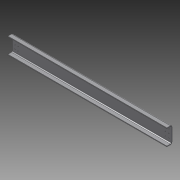
# Autodesk Inventor part: Base Back Bar
Saved by Autodesk Inventor 2012 (Build 160160000, 160)
## iProperties
Created: 2011-10-13
Part Number: Base Back Bar
Material: Default
Document SubType Name: Sheet Metal
Designer: Tushar
Density: 1 g/cm^3
Sheet Metal Rule: Default
Author: Tushar
Autodesk Inventor part; units mm, degrees
ref_plane "YZ Plane" through (0, 0, 0) normal (1, 0, 0) x (0, 1, 0)
ref_plane "XZ Plane" through (0, 0, 0) normal (0, 1, 0) x (-1, 0, 0)
ref_plane "XY Plane" through (0, 0, 0) normal (0, 0, 1) x (1, 0, 0)
sketch "Sketch2" plane through (0, 0, 0) normal (0, 0, 1) x (1, 0, 0)
  line L0 (-301.752, 25.273) -> (301.752, 25.273)
  line L1 (301.752, 25.273) -> (301.752, -25.273)
  line L2 (301.752, -25.273) -> (-301.752, -25.273)
  line L3 (-301.752, -25.273) -> (-301.752, 25.273)
  point P0 (0, 0)
  dimension "d0" = 301.752
  dimension "d1" = 301.752
  dimension "d2" = 25.273
  dimension "d3" = 25.273
  measures "d0" distance from line of L1 point (0, 0)
  measures "d1" distance from line of L3 point (0, 0)
  measures "d2" distance from line of L0 point (0, 0)
  measures "d3" distance from line of L2 point (0, 0)
extrude "Plate1" add sketch "Sketch2" along normal blind 3.048
sketch "Sketch3" plane through (301.752, -25.273, 0) normal (1, 0, 0) x (0, 0, -1)
  line L0 (0, 50.546) -> (-3.048, 50.546)
  arc A0 (0, 50.546) -> (-6.223, 56.769) centre (-6.223, 50.546) ccw
  line L1 (-6.223, 50.546) -> (-6.223, 56.769) construction
  line L2 (-6.223, 50.546) -> (0, 50.546) construction
  line L3 (-6.223, 56.769) -> (-19.5834, 56.769)
  point P0 (0, 25.273)
  dimension "d5" = 90
  dimension "d6" = 6.223
  dimension "d7" = 6.223
  dimension "d8" = 13.3604
  measures "d5" angle of L2 L1
  measures "d6" radius of A0
  measures "d7" distance from line of L0 L1.end
  measures "d8" distance of L1.end L3.end
contour flange "Contour Flange1" sketch "Sketch3" thickness 3.048 bend radius 3.048 curves A0 L3 edges at (0, 25.273, 0) running between points at (-301.752, 25.273, 0) (301.752, 25.273, 0)
bend "Bend1"
corner "Corner1"
sketch "Sketch4" plane through (301.752, -25.273, 3.048) normal (1, 0, 0) x (0, 0, -1)
  line L0 (3.048, 0) -> (0, 0)
  arc A0 (-3.175, -6.223) -> (3.048, 0) centre (-3.175, 0) ccw
  line L1 (-3.175, 0) -> (-3.175, -6.223) construction
  line L2 (-3.175, 0) -> (3.048, 0) construction
  line L3 (-3.175, -6.223) -> (-16.5354, -6.223)
  point P0 (3.048, 25.273)
  dimension "d18" = 90
  dimension "d19" = 6.223
  dimension "d20" = 6.223
  dimension "d21" = 13.3604
  measures "d18" angle of L1 L2
  measures "d19" radius of A0
  measures "d20" distance from line of L0 L1.end
  measures "d21" distance of L1.end L3.end
contour flange "Contour Flange2" sketch "Sketch4" thickness 3.048 bend radius 3.048 curves L3 A0 edges at (0, -25.273, 0) running between points at (301.752, -25.273, 0) (-301.752, -25.273, 0)
bend "Bend2"
corner "Corner2"
sketch "Sketch5" plane through (0, 0, 0) normal (0, 0, -1) x (-1, 0, 0)
  line L0 (-301.752, 25.273) -> (-301.752, -25.273) projected
  line L1 (-301.752, -25.273) -> (301.752, -25.273) projected
  line L2 (301.752, -25.273) -> (301.752, 25.273) projected
  point P0 (0, 0)
  point P1 (-292.354, -15.748)
  point P2 (279.654, -15.748)
  dimension "d31" = 9.398
  dimension "d32" = 22.098
  dimension "d33" = 9.525
  dimension "d34" = 9.525
  measures "d31" distance from line of L0 point (-292.354, -15.748)
  measures "d32" distance from line of L2 point (279.654, -15.748)
  measures "d33" distance from line of L1 point (-292.354, -15.748)
  measures "d34" distance from line of point (279.654, -15.748) L1
hole "Hole1" at (292.354, -15.748, 0) at (-279.654, -15.748, 0) direction (0, 0, 1) diameter 3.175 end through all
sketch "Sketch6" plane through (0, 0, 0) normal (0, 0, -1) x (-1, 0, 0)
  circle A0 centre (-292.354, -15.748) radius 1.5875 projected
  line L0 (301.752, -25.273) -> (301.752, 25.273) projected
  line L1 (-292.354, -15.748) -> (-277.2602, -15.748)
  point P0 (0, 0)
  constraints: 2 end point, 1 perpendicular
sketch "Sketch7" plane through (0, 0, 0) normal (0, 0, -1) x (-1, 0, 0)
  circle A0 centre (-292.354, -15.748) radius 1.5875 projected
  line L0 (301.752, -25.273) -> (301.752, 25.273) projected
  line L1 (-292.354, -15.748) -> (-292.354, -4.4863)
  point P0 (0, 0)
  constraints: 2 end point, 1 parallel
pattern_linear "Rectangular Pattern1" count 2 spacing 12.7 along (-1, 0, 0) count 3 spacing 15.748 along (0, 1, 0) of "Hole1"
equation "\"d34\" = d33"
equation "\"d40\" = Thickness"
equation "\"d9\" = BendReliefWidth"
equation "\"d10\" = BendReliefDepth"
equation "\"d11\" = MinimumRemnant"
equation "\"d12\" = BendRadius"
equation "\"d13\" = BendRadius"
equation "\"d15\" = CornerReliefSize"
equation "\"d16\" = GapSize"
equation "\"d17\" = JacobiRadiusSize"
equation "\"d22\" = BendReliefWidth"
equation "\"d23\" = BendReliefDepth"
equation "\"d24\" = MinimumRemnant"
equation "\"d25\" = BendRadius"
equation "\"d26\" = BendRadius"
equation "\"d28\" = CornerReliefSize"
equation "\"d29\" = GapSize"
equation "\"d30\" = JacobiRadiusSize"
equation "\"d1\" = d0"
equation "\"d3\" = d2"
equation "\"BendRadius\" = Thickness"
equation "\"BendReliefWidth\" = Thickness"
equation "\"BendReliefDepth\" = 0.5 * Thickness"
equation "\"CornerReliefSize\" = 4 * Thickness"
equation "\"MinimumRemnant\" = 2 * Thickness"
equation "\"TransitionRadius\" = BendRadius"
equation "\"JacobiRadiusSize\" = BendRadius"
equation "\"GapSize\" = Thickness"
equation "\"d4\" = BendRadius"
equation "\"Thickness\" = 3.048"
body "Solid1"
